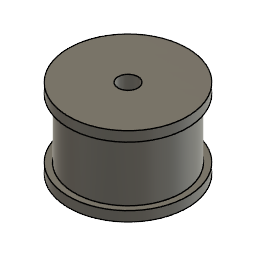
_Pulley Idler HTD 3M x 15.06c5066a-fb81-435f-a3b8-b53ed64e1860 (Autodesk Fusion 360 design; units mm, degrees)
Autodesk Fusion 360 part; units mm, degrees
sketch "Sketch1" plane through (0, 0, 0) normal (0, 1, 0) x (1, 0, 0)
  circle A0 centre (0, 0) radius 2.5
  circle A1 centre (0, 0) radius 13.5
  circle A2 centre (0, 0) radius 15
  dimension "d1" = 5
  dimension "d2" = 27
  constraint coincident A0.centre A1.centre
  measures "d1" diameter of A0
  measures "d2" diameter of A1
extrude "Extrude1" add sketch "Sketch1" against normal blind 2.5 contours A1 | A2
extrude "Extrude2" add sketch "Sketch1" along normal blind 15 contours A1
extrude "Extrude3" add sketch "Sketch1" along normal blind 2.5 from surface at 15 contours A1 | A2
